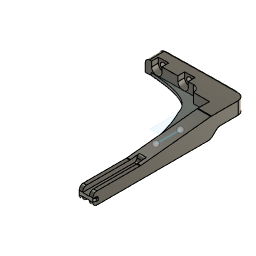
Long_Narrow_Gripper_Extended v1 (Autodesk Fusion 360 design; units mm, degrees)
Autodesk Fusion 360 part; units mm, degrees
note: some values were not read from the file. Chosen so that the rebuilt part matches the saved one: which bodies a step acts on; which face or edge a step refers to; which pieces of a blend or face edit are solid. Set by a fixed rule: which sketch regions a step uses.
sketch "Sketch1" plane through (0, 0, 0) normal (0, 0, 1) x (1, 0, 0)
  line L0 (49.9924, -0.8726) -> (0, 0)
  line L1 (0, 0) -> (0, -112)
  line L2 (0, -112) -> (10, -112)
  line L3 (10, -112) -> (10, -11.1762)
  line L4 (10, -11.1762) -> (49.8004, -11.8709)
  line L5 (49.8004, -11.8709) -> (49.9924, -0.8726)
  dimension "d3" = 11
  dimension "d4" = 10
  dimension "d54" = 112
  dimension "d67" = 50
  dimension "d68" = 89
  constraint perpendicular L2 L3
  constraint parallel L0 L4
  constraint perpendicular L0 L5
  constraint coincident L0.end L1.start
  constraint coincident L1.end L2.start
  constraint vertical L1
  constraint horizontal L2
  measures "d3" distance of L0.start L4.end
  measures "d4" distance of L1.end L2.end
  measures "d54" distance of L0.end L2
  measures "d67" distance of L0.start L0.end
  measures "d68" angle of L0 L1
extrude "Extrude1" add sketch "Sketch1" along normal blind 14.5 makes body 1
sketch "Sketch2" plane through (0, 0, 0) normal (1, 0, 0) x (0, 1, 0)
  line L0 (0, 0) -> (0, 9.25)
  line L1 (0, 9.25) -> (-20, 9.25)
  line L2 (-20, 9.25) -> (-25.25, 14.5)
  line L3 (-25.25, 14.5) -> (-112, 14.5)
  line L4 (-112, 14.5) -> (-112, 5.5)
  line L5 (-112, 5.5) -> (-77, 5.5)
  line L6 (-77, 5.5) -> (-25, 0)
  line L7 (-25, 0) -> (0, 0)
  dimension "d7" = 9.25
  dimension "d8" = 9
  dimension "d9" = 135
  dimension "d11" = 20
  dimension "d69" = 35
  dimension "d70" = 25
  dimension "d73" = 5.25
  dimension "d74" = 112
  constraint coincident L0.start L7.end
  constraint vertical L0
  constraint perpendicular L0 L1
  constraint horizontal L3
  constraint perpendicular L3 L4
  constraint perpendicular L4 L5
  constraint perpendicular L0 L7
  measures "d7" distance of L0.start L0.end
  measures "d8" distance of L3.end L4.end
  measures "d9" angle of L1 L2
  measures "d11" distance of L0.end L1.end
  measures "d69" distance of L4.end L5.end
  measures "d70" distance of L6.end L0.start
  measures "d73" distance of L1 L3
  measures "d74" distance of L0 L4
surface "Extrude2" add extruded along (1, 0, 0) between 0 and 55 profiles "Sketch2" section 1 separate body makes body 2
split "Split1" by bodies 2 bodies 1 makes body 3 at (19.9975, -4.0163, 14.5) makes body 4 at (6.6667, -54, 0)
delete_body "RemoveBody1" bodies 3
delete_body "RemoveBody2" bodies 4
delete_body "RemoveBody3" bodies 2
ref_plane "WorkPlane3" through (29.9002, -11.5236, 7.25) normal (-0.017452, -0.999848, 0) x (0.999848, -0.017452, 0)
sketch "Sketch4" plane through (29.9002, -11.5236, 4.75) normal (-0.017452, -0.999848, 0) x (0.999848, -0.017452, 0)
  line L0 (-19.9032, -4.75) -> (19.9032, -4.75)
  line L1 (-19.9032, -4.75) -> (-19.9032, 4.5)
  line L2 (-11.1532, -1) -> (-11.1532, -4.75)
  line L3 (-3.6532, -1) -> (-3.6532, -4.75)
  line L4 (-11.1532, -4.75) -> (-3.6532, -4.75)
  arc A0 (-3.6532, -1) -> (-11.1532, -1) centre (-7.4032, -1) ccw
  line L5 (15.3468, -1) -> (15.3468, -4.75)
  line L6 (7.8468, -1) -> (7.8468, -4.75)
  arc A1 (15.3468, -1) -> (7.8468, -1) centre (11.5968, -1) ccw
  line L7 (7.8468, -4.75) -> (15.3468, -4.75)
  dimension "d19" = 7.5
  dimension "d21" = 12.5
  dimension "d24" = 19
  dimension "d25" = 0
  constraint tangent L0 A0
  constraint coincident L0 L2.end
  constraint tangent L2 A0
  constraint perpendicular L0 L2
  constraint coincident L0 L3.end
  constraint tangent L3 A0
  constraint perpendicular L0 L3
  measures "d19" diameter of A0
  measures "d21" distance of A0.centre L1
extrude "Extrude4" cut sketch "Sketch4" against normal blind 5 bodies 1
sketch "Sketch5" plane through (29.9002, -11.5236, 4.75) normal (-0.017452, -0.999848, 0) x (0.999848, -0.017452, 0)
  circle A0 centre (-7.4032, -1) radius 2.25
  arc A1 (-3.6532, -1) -> (-11.1532, -1) centre (-7.4032, -1) ccw
  circle A2 centre (11.5968, -1) radius 2.25
  arc A3 (15.3468, -1) -> (7.8468, -1) centre (11.5968, -1) ccw
  dimension "d28" = 4.5
  constraint concentric A0 A1
  constraint concentric A2 A3
  constraint equal A0 A2
  measures "d28" diameter of A0
extrude "Extrude5" cut sketch "Sketch5" against normal through all bodies 1
ref_plane "WorkPlane4" through (24.9962, -0.4363, 7.25) normal (0.017452, 0.999848, 0) x (-0.999848, 0.017452, 0)
sketch "Sketch6" plane through (24.9962, -0.4363, 4.75) normal (0.017452, 0.999848, 0) x (-0.999848, 0.017452, 0)
  line L0 (-25, -4.75) -> (25, -4.75) construction
  line L1 (-25, -4.75) -> (-25, 4.5) construction
  line L2 (-25, 4.5) -> (19, 4.5)
  line L3 (19, 4.5) -> (19, 1.35)
  line L4 (19, 1.35) -> (-25, 1.35)
  line L5 (-25, 1.35) -> (-25, 4.5)
  line L6 (-22, -4.75) -> (19, -4.75)
  line L7 (19, -4.75) -> (19, -3.35)
  line L8 (19, -3.35) -> (-22, -3.35)
  line L9 (-22, -3.35) -> (-22, -4.75)
  circle A0 centre (-16.6935, -1) radius 2.25 construction
  circle A1 centre (2.3065, -1) radius 2.25 construction
  line L10 (-16.6935, -1) -> (2.3065, -1) construction
  line L11 (25, -4.75) -> (25, 4.5)
  dimension "d32" = 4.7
  dimension "d47" = 3
  dimension "d72" = 6
  constraint horizontal L2
  constraint horizontal L4
  constraint horizontal L6
  constraint horizontal L8
  constraint coincident A0.centre L10.start
  constraint coincident A1.centre L10.end
  constraint coincident L4.start L3
  constraint perpendicular L3 L4
  constraint coincident L7.end L8.start
  constraint collinear L3 L7
  constraint coincident L1.end L2.start
  constraint vertical L5
  measures "d32" distance of L4 L8
  measures "d47" distance of L1 L9
  measures "d72" distance of L3 L11
extrude "Extrude6" add sketch "Sketch6" along normal blind 0.6 draft -30 bodies 1
ref_plane "WorkPlane1" through (5, -68.625, 10) normal (0, 0, 1) x (1, 0, 0)
ref_plane "WorkPlane2" through (0, -112, 0) normal (0, 1, 0) x (0, 0, 1)
sketch "Sketch3" plane through (5, -68.5, 10) normal (0, 0, 1) x (1, 0, 0)
  line L0 (-5, -43.5) -> (-6, -42)
  line L1 (-6, -42) -> (-6, -40.5)
  line L2 (-6, -40.5) -> (6, -40.5)
  line L3 (6, -40.5) -> (6, -42)
  line L4 (6, -42) -> (5, -43.5)
  line L5 (5, -43.5) -> (-5, -43.5)
  constraint vertical L1
  constraint perpendicular L1 L2
  constraint perpendicular L2 L3
  constraint perpendicular L3 L5
extrude "Extrude3" add sketch "Sketch3" along normal mid plane 2 bodies 1
sketch "Sketch7" plane through (5, -112, 10) normal (0, 1, 0) x (1, 0, 0)
  line L0 (2.5, 6.25) -> (-2.5, 6.25)
  line L1 (-2.5, 6.25) -> (-2.5, 1.25)
  line L2 (-2.5, 1.25) -> (2.5, 1.25)
  line L3 (2.5, 1.25) -> (2.5, 6.25)
  line L4 (2.5, 6.25) -> (-2.5, 1.25) construction
  line L5 (-2.5, 6.25) -> (2.5, 1.25) construction
  line L6 (-10, 0) -> (10, 0) construction
  line L7 (2.5, -6.25) -> (-2.5, -6.25)
  line L8 (-2.5, -6.25) -> (2.5, -1.25) construction
  line L9 (-2.5, -6.25) -> (-2.5, -1.25)
  line L10 (2.5, -6.25) -> (-2.5, -1.25) construction
  line L11 (-2.5, -1.25) -> (2.5, -1.25)
  line L12 (2.5, -1.25) -> (2.5, -6.25)
  point P0 (0, 3.75)
  point P1 (0, -3.75)
  dimension "d39" = 5
  dimension "d40" = 5
  dimension "d41" = 2.5
  constraint horizontal L0
  constraint perpendicular L0 L1
  constraint parallel L0 L2
  constraint parallel L1 L3
  constraint coincident L4 P0
  constraint coincident L5 P0
  constraint perpendicular L1 L6
  constraint symmetric L0.start L6 L7.start
  constraint symmetric L0.end L6 L7.end
  constraint symmetric L1.end L6 L9.end
  constraint symmetric L2.end L6 L8.end
  constraint symmetric P0 L6 P1
  measures "d39" distance of L1.end L2.end
  measures "d40" distance of L0.end L1.end
  measures "d41" distance of L2 L11
extrude "Extrude7" cut sketch "Sketch7" along normal blind 40 contours L0 L1 L2 L3 bodies 1
extrude "Extrude8" cut sketch "Sketch7" along normal blind 40 contours L7 L9 L11 L12 bodies 1
fillet "Fillet3" radius 2 4 edges at (5, -72, 11.25) (5, -72, 14.5) (5, -72, 8.75) (5, -72, 4.9712) on bodies 1
ref_plane "WorkPlane5" through (24.9962, -10, 9.25) normal (0, 0, 1) x (0, -1, 0)
sketch "Sketch8" plane through (19.5408, -8.9645, 9.25) normal (0, 0, 1) x (1, 0, 0)
  line L0 (26.0328, -2.8327) -> (-9.5408, -2.2118)
  line L1 (-9.5408, -18.3566) -> (-9.5408, -2.2118)
  spline S0 degree 5 poles (-9.5408, -18.3566) (-9.3855, -17.7813) (-9.0214, -16.6561) (-8.315, -15.0447) (-7.0468, -13.0515) (-4.887, -10.8335) (-2.1191, -8.9052) (1.2711, -7.2732) (5.2484, -5.9208) (9.7561, -4.821) (14.7357, -3.9458) (19.0585, -3.4073) (22.4779, -3.0877) (24.8349, -2.9115) (26.0328, -2.8327) knots 0 0 0 0 0 0 0.1 0.2 0.3 0.4 0.5 0.6 0.7 0.8 0.9 1 1 1 1 1 1
  line L2 (-9.5408, -2.2118) -> (30.2596, -2.9065)
  point P0 (-2, -9)
  constraint coincident L0.end L1.end
  constraint coincident L1.start S0.start
  constraint collinear L0 L2
  constraint vertical L1
extrude "Extrude9" add sketch "Sketch8" against normal blind 2 bodies 1
fillet "Fillet1" radius 5 5 edges at (5, -20, 9.25) (5, -25.25, 14.5) (1.25, -77, 5.5) (8.75, -77, 5.5) (5, -25, 0) on bodies 1
fillet "Fillet2" radius 3 12 edges at (10, -112, 7.25) (10, -112, 12.75) (0, -112, 7.25) (0, -112, 12.75) (8.75, -112, 5.5) (7.5, -112, 7.125) (2.5, -112, 7.125) (1.25, -112, 5.5) (1.25, -112, 14.5) (2.5, -112, 12.875) (7.5, -112, 12.875) (8.75, -112, 14.5) on bodies 1
fillet "Fillet5" radius 3 1 edges at (49.8964, -6.3718, 0) on bodies 1
fillet "Fillet8" radius 5 2 edges at (0, 0, 4.625) (10, -11.1762, 3.625) on bodies 1
move_body "Move1" bodies 1 to x (-1, 0, 0) y (0, 1, 0) z (0, 0, -1) at (0, 0, 0)
sketch "Sketch9" plane through (0, 0, 0) normal (0, 0, 1) x (-1, 0, 0)
  arc A0 (0, 5.088) -> (5.0873, 0.0888) centre (5, 5.088) ccw
  line L0 (5.0873, 0.0888) -> (5.9991, 0.1047)
  line L1 (5.9991, 0.1047) -> (46.9928, 0.8203)
  line L2 (46.9928, 0.8203) -> (46.8009, 11.8186)
  line L3 (46.8009, 11.8186) -> (45.2446, 11.7914)
  line L4 (45.2446, 11.7914) -> (45.3319, 6.7922)
  line L5 (45.3319, 6.7922) -> (37.833, 6.6613)
  line L6 (37.833, 6.6613) -> (37.7458, 11.6605)
  line L7 (37.7458, 11.6605) -> (26.2475, 11.4598)
  line L8 (26.2475, 11.4598) -> (26.3348, 6.4606)
  line L9 (26.3348, 6.4606) -> (18.8359, 6.3297)
  line L10 (18.8359, 6.3297) -> (18.7487, 11.3289)
  line L11 (18.7487, 11.3289) -> (15.0873, 11.265)
  arc A1 (10, 16.2643) -> (15.0873, 11.265) centre (15, 16.2643) ccw
  line L12 (10, 16.2643) -> (10, 24.7363)
  line L13 (10, 24.7363) -> (0, 24.7363)
  line L14 (0, 24.7363) -> (0, 5.088)
  line L15 (10, 8) -> (10, 16.2643)
  line L16 (10, 16.3682) -> (10, 24.7363)
  line L17 (10, 8) -> (10, 6)
  line L18 (10, 6) -> (10, 3)
  constraint coincident L12.end L13.start
  constraint coincident A1.start L12.start
  constraint tangent A1 L15
  constraint parallel L15 L17
  constraint parallel L17 L18
split "Split2" by curves path "Sketch9" along L18 L17 L15 bodies 1 makes body 5 at (-10.3333, -111.5, -10.3333) makes body 6 at (-30.8133, -4.7723, -9.25)
move_body "Move2" bodies 6 to x (1, 0, 0) y (0, 1, 0) z (0, 0, 1) at (-11.7375, -0.3475, 0)
extrude "Extrude10" add 5 faces at (-21.7375, -11.1022, -5.5) (-21.7375, -7.6808, -6.1667) (-21.7375, -5.3475, -6.1667) (-21.7375, -2.4057, -5.1167) (-21.7375, -20.8522, -7.9167) along direction (1, 0, 0) blind 10 on bodies 6 bodies 6
extrude "Extrude11" add 1 faces at (-11.7375, -11.2485, -2.8833) along direction (1, 0, 0) blind 1.5 on bodies 6 bodies 6
move_body "Move3" bodies 1 to x (1, 0, 0) y (0, 1, 0) z (0, 0, 1) at (0, -0.35, 0)
extrude "Extrude12" add 1 faces at (-10.2375, -11.2485, -2.8833) along direction (1, 0, 0) blind 0.5 on bodies 6 bodies 6 5 1
sketch "Sketch10" plane through (0, -27.6686, 0) normal (0, -1, 0) x (1, 0, 0)
  line L0 (-21.7375, -7.25) -> (-21.7375, -9.25)
  line L1 (-21.7375, -9.25) -> (-10, -9.25)
  line L2 (-10, -9.25) -> (-10, -7.25)
  line L3 (-10, -7.25) -> (-21.7375, -7.25)
extrude "Extrude13" add sketch "Sketch10" along normal blind 21 bodies 6
sketch "Sketch11" plane through (0, 0, -7.25) normal (0, 0, 1) x (-1, 0, 0)
  arc A0 (21.7375, 16.6118) -> (26.8247, 11.6125) centre (26.7375, 16.6118) ccw
  line L0 (26.8247, 11.6125) -> (32.8895, 11.7184)
  line L1 (32.8895, 11.7184) -> (35.5816, 11.7654)
  line L2 (35.5816, 11.7654) -> (51.8866, 12.05)
  line L3 (51.8866, 12.05) -> (54.5787, 12.097)
  line L4 (54.5787, 12.097) -> (57.311, 12.1447)
  spline S0 degree 5 poles (57.311, 12.1447) (56.1132, 12.2235) (53.7561, 12.3997) (50.3368, 12.7192) (46.0139, 13.2578) (41.0343, 14.1329) (36.5266, 15.2328) (32.5493, 16.5852) (29.1591, 18.2172) (26.3912, 20.1455) (24.2314, 22.3634) (22.9633, 24.3566) (22.2568, 25.968) (21.8927, 27.0932) (21.7375, 27.6686) knots -1 -1 -1 -1 -1 -1 -0.9 -0.8 -0.7 -0.6 -0.5 -0.4 -0.3 -0.2 -0.1 0 0 0 0 0 0
  line L5 (21.7375, 27.6686) -> (21.7375, 48.6686)
  line L6 (21.7375, 48.6686) -> (10, 48.6686)
  line L7 (10, 48.6686) -> (10, 16.6118)
  line L8 (10, 16.6118) -> (21.7375, 16.6118)
extrude "Extrude14" add 1 faces at (-13.9125, -48.6686, -8.5833) along direction (0, -1, 0) blind 30 on bodies 6 bodies 6
sketch "Sketch12" plane through (0, 0, -7.25) normal (0, 0, 1) x (-1, 0, 0)
extrude "Extrude15" add 1 faces at (-13.9125, -78.6686, -8.5833) along direction (0, -1, 0) blind 20 on bodies 6 bodies 6
sketch "Sketch13" plane through (0, 0, -7.25) normal (0, 0, 1) x (-1, 0, 0)
  arc A0 (21.7375, 16.6118) -> (26.8247, 11.6125) centre (26.7375, 16.6118) ccw
  line L0 (26.8247, 11.6125) -> (32.8895, 11.7184)
  line L1 (32.8895, 11.7184) -> (35.5816, 11.7654)
  line L2 (35.5816, 11.7654) -> (51.8866, 12.05)
  line L3 (51.8866, 12.05) -> (54.5787, 12.097)
  line L4 (54.5787, 12.097) -> (57.311, 12.1447)
  spline S0 degree 5 poles (57.311, 12.1447) (56.1132, 12.2235) (53.7561, 12.3997) (50.3368, 12.7192) (46.0139, 13.2578) (41.0343, 14.1329) (36.5266, 15.2328) (32.5493, 16.5852) (29.1591, 18.2172) (26.3912, 20.1455) (24.2314, 22.3634) (22.9633, 24.3566) (22.2568, 25.968) (21.8927, 27.0932) (21.7375, 27.6686) knots -1 -1 -1 -1 -1 -1 -0.9 -0.8 -0.7 -0.6 -0.5 -0.4 -0.3 -0.2 -0.1 0 0 0 0 0 0
  line L5 (21.7375, 27.6686) -> (21.7375, 98.6686)
  line L6 (21.7375, 98.6686) -> (10, 98.6686)
  line L7 (10, 98.6686) -> (10, 16.6118)
  line L8 (10, 16.6118) -> (21.7375, 16.6118)
  spline S1 degree 5 poles (21.7375, 27.6686) (21.2399, 28.6481) (20.2693, 30.6479) (18.8865, 33.7704) (17.1914, 38.1829) (15.3357, 44.1398) (13.7616, 50.5685) (12.483, 57.4927) (11.4933, 64.9012) (10.7691, 72.755) (10.2846, 81.0103) (10.0703, 87.9051) (10.0004, 93.2286) (9.9935, 96.8441) (10, 98.6686) knots 0 0 0 0 0 0 0.1 0.2 0.3 0.4 0.5 0.6 0.7 0.8 0.9 1 1 1 1 1 1
  point P0 (13.3452, 53.1051)
  constraint coincident S0.end L5.start
  constraint coincident L6.end L7.start
split "Split3" by curves path "Sketch13" along S1 bodies 6 makes body 7 at (-48.849, -4.949, -9.25) makes body 8 at (-14.4404, -86.3906, -7.25)
move_body "Move4" bodies 8 to x (1, 0, 0) y (0, 1, 0) z (0, 0, 1) at (-19.6656, 1.5193, 2.2375)
delete_body "RemoveBody4" bodies 8
combine "Combine1" operation add target body 6 tool bodies 7
combine "Combine2" operation add target body 6 tool bodies 5
copy_body "CopyPasteBodies1" bodies 6 makes body 9
move_body "Move5" bodies 9 to x (-1, 0, 0) y (0, 1, 0) z (0, 0, -1) at (-88.5792, -0.0849, -23.6183)
move_body "Move6" bodies 9 to x (1, 0, 0) y (0, 1, 0) z (0, 0, 1) at (0.0069, 0.2339, 3.9688)
delete_body "RemoveBody5" bodies 9
sketch "Sketch14" plane through (0, 0, -7.25) normal (0, 0, 1) x (-1, 0, 0)
  line L0 (10, 38) -> (10, 56)
  constraint vertical L0
